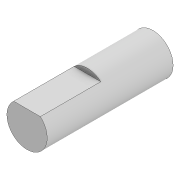
# Autodesk Inventor part: shaft
Saved by Autodesk Inventor 2020 (Build 240168000, 168)
## iProperties
Created: 2020-08-28
Part Number: shaft
Material: 일반
Document SubType Name: Modeling
Designer: 이호석
Mass: 1.21312 g
Surface Area: 7.22965 cm^2
Volume: 1.21312 cm^3
Density: 1 g/cm^3
Appearance: 기본값
Author: 이호석
Autodesk Inventor part; units mm, degrees
ref_plane "YZ Plane" through (0, 0, 0) normal (1, 0, 0) x (0, 1, 0)
ref_plane "XZ Plane" through (0, 0, 0) normal (0, 1, 0) x (-1, 0, 0)
ref_plane "XY Plane" through (0, 0, 0) normal (0, 0, 1) x (1, 0, 0)
sketch "스케치1" plane through (0, 0, 0) normal (0, 0, 1) x (1, 0, 0)
  circle A0 centre (0, 0) radius 4
  dimension "d0" = 8
  constraints: 1 centre point, 1 coincident
  measures "d0" diameter of A0
extrude "돌출1" add sketch "스케치1" along normal blind 25
sketch "스케치2" plane through (0, 0, 25) normal (0, 0, 1) x (1, 0, 0)
  circle A0 centre (0, 0) radius 4 projected
  line L0 (0, -4) -> (0, 3)
  line L1 (2.6458, 3) -> (-2.6458, 3)
  dimension "d3" = 7
  constraints: 4 end point, 3 point on circle, 1 horizontal, 1 vertical
  measures "d3" distance of L0.start L0.end
extrude "돌출2" cut sketch "스케치2" against normal blind 12 contours L1 A0
